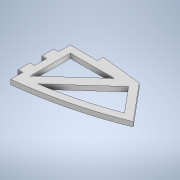
# Autodesk Inventor part: bulkhead_F2
Saved by Autodesk Inventor 2020.3 (Build 243373000, 373)
## iProperties
Created: 2020-05-22
Part Number: bulkhead_F2
Material: Generic
Document SubType Name: Modeling
Designer: kardo
Density: 1 g/cm^3
Appearance: Default
Mass: 0.941689 g
Surface Area: 14.623 cm^2
Volume: 0.941689 cm^3
Author: kardo
Autodesk Inventor part; units mm, degrees
ref_plane "YZ Plane" through (0, 0, 0) normal (1, 0, 0) x (0, 1, 0)
ref_plane "XZ Plane" through (0, 0, 0) normal (0, 1, 0) x (-1, 0, 0)
ref_plane "XY Plane" through (0, 0, 0) normal (0, 0, 1) x (1, 0, 0)
derived "base_sketch.ipt"
sketch "bulkhead_F2" plane through (0, 158.1, 32.9472) normal (0, 1, 0) x (-1, 0, 0)
  line L0 (19.176, 13.8708) -> (62.322, 13.8708)
  line L1 (62.322, 13.8708) -> (62.322, -19.7029)
  line L2 (0, -32.9472) -> (-11.5056, -32.9472)
  line L3 (-11.5056, -35.434) -> (-34.5168, -32.9472)
  line L4 (-11.5056, -32.9472) -> (-11.5056, -35.434)
  line L5 (-34.5168, -32.9472) -> (-57.528, -5.4072)
  line L6 (0, 6.0797) -> (0, -19.2614)
  line L7 (0, -19.2614) -> (-11.5056, -19.2614)
  line L8 (-11.5056, -19.2614) -> (-11.5056, -21.7481)
  line L9 (-11.5056, -21.7481) -> (-28.7096, -19.8889)
  line L10 (-28.7096, -19.8889) -> (-41.6391, -4.4149)
  line L11 (-57.528, -12.2803) -> (-57.528, -5.4072) construction
  line L12 (-38.352, 3.7728) -> (-38.352, -3.1003) construction
  line L13 (-19.176, 9.648) -> (-19.176, 2.7749) construction
  line L14 (0, 12.9528) -> (0, 6.0797) construction
  line L15 (-57.528, -7.15) -> (0, 2.7528) construction
  spline S0 degree 4 poles (-57.528, -5.4072) (-46.0483, 1.2579) (-30.6129, 7.5809) (-11.2214, 12.0942) (8.3201, 13.8708) (15.5662, 13.8708) (19.176, 13.8708) knots 0 0 0 0 0 0.630279 0.815816 1 1 1 1 1
  spline S1 degree 3 poles (-57.528, -12.2803) (-39.18, -1.6112) (-19.6272, 3.8157) (0, 6.0797) knots 0 0 0 0 1 1 1 1
ref_plane "bulkhead_F2_plane" through (0, 158.1, 32.9472) normal (0, 1, 0) x (-1, 0, 0)
sketch "Sketch2" plane through (0, 158.1, 32.9472) normal (0, 1, 0) x (-1, 0, 0)
  spline S0 degree 3 poles (-57.528, -12.2803) (-39.18, -1.6112) (-19.6272, 3.8157) (0, 6.0797) knots 0 0 0 0 1 1 1 1 projected
  line L0 (-28.7096, -19.8889) -> (-41.6391, -4.4149) projected
  line L1 (-11.5056, -21.7481) -> (-28.7096, -19.8889) projected
  line L2 (-11.5056, -19.2614) -> (-11.5056, -21.7481) projected
  line L3 (0, -19.2614) -> (-11.5056, -19.2614) projected
  line L4 (-36.6789, -5.6724) -> (-27.7664, -16.339)
  line L5 (-27.7664, -16.339) -> (-7.4667, 2.0227)
  line L6 (-28.7096, -19.8889) -> (0, 6.0797) construction
  line L7 (-21.7177, -16.2614) -> (-3, -16.2614)
  line L8 (-3, -16.2614) -> (-3, 0.6693)
  line L9 (-3, 0.6693) -> (-21.7177, -16.2614)
  line L10 (0, 1.0115) -> (2, 1.0115)
  line L11 (2, 1.0115) -> (2, -4.0567)
  line L12 (2, -4.0567) -> (0, -4.0567)
  line L13 (0, -9.125) -> (2, -9.125)
  line L14 (2, -9.125) -> (2, -14.1932)
  line L15 (2, -14.1932) -> (0, -14.1932)
  spline S1 degree 2 poles (-36.6789, -5.6724) (-22.4646, -0.3374) (-7.4667, 2.0227) knots 0 0 0 1 1 1
  line L16 (-36.6789, -5.6724) -> (-37.7437, -2.8677) construction
  line L17 (-22.2687, -1.0812) -> (-23.0275, 1.8213) construction
  line L18 (-7.4667, 2.0227) -> (-7.9439, 4.9845) construction
  line L19 (-36.6789, -5.6724) -> (-22.2687, -1.0812) construction
  line L20 (-22.2687, -1.0812) -> (-7.4667, 2.0227) construction
  line L21 (0, 1.0115) -> (0, 6.0797)
  line L22 (0, -4.0567) -> (0, -9.125)
  line L23 (0, -14.1932) -> (0, -19.2614)
  point P0 (0, -32.9472)
  dimension "d1" = 4
  dimension "d2" = 3
  dimension "d4" = 3
  dimension "d5" = 3
  dimension "d6" = 2
  dimension "d7" = 3
  constraints: 40 end point, 7 equal length, 4 collinear, 4 horizontal, 4 parallel, 2 vertical, 10 other
  measures "d1" distance between parallel lines of L9 L5
  measures "d2" distance between parallel lines of L3 L7
  measures "d4" distance between parallel lines of L0 L4
  measures "d5" distance of L4.start L16.end
  measures "d6" distance of L14.end L15.end
  measures "d7" distance between parallel lines of L22 L8
extrude "Extrusion1" add sketch "Sketch2" along normal blind 2
equation "\"d6\" = stringer_thickness"
equation "\"d8\" = bulkhead_thickness"
equation "\"stringer_thickness\" = 2"
equation "\"bulkhead_thickness\" = 2"
body "Solid1"
